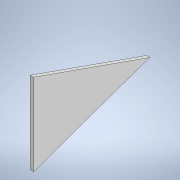
# Autodesk Inventor part: Part2
Saved by Autodesk Inventor 2022.2 (Build 262287000, 287)
## iProperties
Created: 2022-02-28
Part Number: Part2
Material: Generic
Document SubType Name: Modeling
Designer: PRASHANTH
Density: 1 g/cm^3
Appearance: Default
Author: PRASHANTH
Autodesk Inventor part; units mm, degrees
ref_plane "YZ Plane" through (0, 0, 0) normal (1, 0, 0) x (0, 1, 0)
ref_plane "XZ Plane" through (0, 0, 0) normal (0, 1, 0) x (-1, 0, 0)
ref_plane "XY Plane" through (0, 0, 0) normal (0, 0, 1) x (1, 0, 0)
sketch "Sketch1" plane through (0, 0, 0) normal (1, 0, 0) x (0, 1, 0)
  line L0 (60, 85) -> (-60, 85)
  line L1 (60, 85) -> (0, -85)
  line L2 (-60, 85) -> (0, -85)
  point P0 (0, 0)
  constraints: 6 end point, 1 horizontal
extrude "Extrusion1" add sketch "Sketch1" along normal blind 5
body "Solid1"
